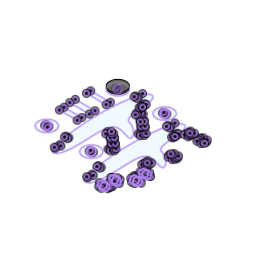
laserbíll (Autodesk Fusion 360 design; units mm, degrees)
Autodesk Fusion 360 part; units mm, degrees
note: some values were not read from the file. Chosen so that the rebuilt part matches the saved one: which bodies a step acts on; which face or edge a step refers to. Set by a fixed rule: which sketch regions a step uses.
(part 1 of 2)
sketch "Sketch2" plane through (0, 0, 0) normal (1, 0, 0) x (0, 1, 0)
  line L0 (0, 0) -> (0, 3) construction
  line L1 (0, 3) -> (-40, 3) construction
  line L2 (-40, 3) -> (-160.4178, 3) construction
  line L3 (-14.8797, 3) -> (-11.8797, 3)
  line L4 (-11.8797, 3) -> (-11.8797, -3)
  line L5 (-14.8797, -3) -> (-14.8797, 3)
  spline S0 degree 5 poles (0, 0) (-0.4976, -0.0964) (-1.4854, -0.3042) (-2.945, -0.6607) (-4.8535, -1.2067) (-7.2026, -1.9204) (-9.0712, -2.4375) (-10.4741, -2.7532) (-11.4109, -2.9243) (-11.8797, -3) knots 0 0 0 0 0 0 0.2 0.4 0.6 0.8 1 1 1 1 1 1
  line L6 (1.6866, 0.3268) -> (-1.6866, -0.3268)
  line L7 (-10.2925, -2.7437) -> (-13.4669, -3.2563)
  line L8 (-160.4178, 3) -> (-163.4178, 3)
  line L9 (-163.4178, 3) -> (-163.4178, -3)
  line L10 (-160.4178, -3) -> (-160.4178, 3)
  spline S1 degree 5 poles (-14.8797, -3) (-22.3096, -4.1508) (-36.7037, -6.1171) (-56.899, -8.0619) (-81.4164, -8.9223) (-109.3682, -8.0716) (-130.3752, -6.4401) (-145.595, -4.8529) (-155.5147, -3.6429) (-160.4178, -3) knots 0 0 0 0 0 0 0.2 0.4 0.6 0.8 1 1 1 1 1 1
  line L11 (2.0883, -0.3719) -> (-31.8477, -5.6281)
  line L12 (-149.202, -4.4707) -> (-171.6337, -1.5293)
  spline S2 degree 5 poles (0, 0) (1.0214, 1.1786) (2.8685, 3.4561) (5.0525, 6.633) (6.7903, 10.3902) (7.0201, 14.2972) (5.3558, 17.4431) (1.9, 19.8865) (-3.1724, 21.7265) (-9.6182, 23.091) (-17.1297, 24.1256) (-25.3371, 24.9813) (-33.8146, 25.8044) (-42.0773, 26.723) (-49.6078, 27.8419) (-55.9536, 29.2551) (-60.806, 31.0538) (-64.092, 33.3377) (-66.0502, 36.222) (-67.344, 39.8538) (-68.8404, 44.3379) (-71.3179, 49.6389) (-75.2304, 55.5069) (-80.3697, 61.3547) (-85.9901, 66.3649) (-91.1225, 69.6901) (-94.8388, 70.6334) (-96.5098, 68.8155) (-96.1359, 64.402) (-94.2949, 58.0341) (-91.8952, 50.6114) (-89.9846, 43.1151) (-89.5511, 36.4298) (-91.2912, 31.1286) (-95.5355, 27.4211) (-102.3274, 25.2561) (-111.4597, 24.382) (-122.527, 24.4246) (-134.9716, 24.9543) (-148.1309, 25.5642) (-161.285, 25.924) (-173.707, 25.7763) (-184.7129, 24.9433) (-193.7115, 23.3296) (-200.2539, 20.9266) (-204.0865, 17.8175) (-205.1955, 14.1795) (-203.8722, 10.294) (-200.7195, 6.5331) (-196.466, 3.2637) (-191.8243, 0.7734) (-187.3088, -0.8279) (-183.1451, -1.6443) (-179.3481, -1.905) (-175.7677, -1.905) (-172.1417, -1.9268) (-168.9623, -2.1457) (-166.3081, -2.4941) (-164.4038, -2.8164) (-163.4178, -3) knots 0 0 0 0 0 0 0.018182 0.036364 0.054545 0.072727 0.090909 0.109091 0.127273 0.145455 0.163636 0.181818 0.2 0.218182 0.236364 0.254545 0.272727 0.290909 0.309091 0.327273 0.345455 0.363636 0.381818 0.4 0.418182 0.436364 0.454545 0.472727 0.490909 0.509091 0.527273 0.545455 0.563636 0.581818 0.6 0.618182 0.636364 0.654545 0.672727 0.690909 0.709091 0.727273 0.745455 0.763636 0.781818 0.8 0.818182 0.836364 0.854545 0.872727 0.890909 0.909091 0.927273 0.945455 0.963636 0.981818 1 1 1 1 1 1
  line L13 (-191.6536, 2.2585) -> (-135.1821, -8.2585)
  line L14 (-184.1519, 9.7365) -> (-194, 8)
  line L15 (-194, 8) -> (-193.4791, 5.0456)
  line L16 (-193.4791, 5.0456) -> (-183.631, 6.7821)
  line L17 (-183.631, 6.7821) -> (-184.1519, 9.7365)
  point P0 (4.968, 17.2018)
  point P1 (-31.0209, 25.5436)
  point P2 (-64.1497, 33.8854)
  point P3 (-72.7298, 51.5223)
  point P4 (-95.1335, 69.6359)
  point P5 (-90, 40)
  point P6 (-131.599, 24.8286)
  point P7 (-204.5301, 15.0567)
  point P8 (-193.3805, 1.7277)
  point P9 (-177.8679, -1.8848)
  dimension "d4" = 3
  dimension "d5" = 3
  dimension "d7" = 3
  dimension "d17" = 6
  dimension "d18" = 6
  dimension "d19" = 6
  dimension "d20" = 6
  dimension "d97" = 10
  dimension "d98" = 3
  constraint coincident L0.start S0.start
  constraint vertical L0
  constraint perpendicular L0 L1
  constraint perpendicular L0 L2
  constraint horizontal L3
  constraint vertical L4
  constraint vertical L5
  constraint coincident L1 L3.start
  constraint midpoint L0.start L6
  constraint midpoint L4.end L7
  constraint horizontal L8
  constraint vertical L9
  constraint vertical L10
  constraint midpoint L5.start L11
  constraint midpoint L10.start L12
  constraint midpoint L9.end L13
  measures "d4" distance of L0.start L0.end
  measures "d5" distance of L3.start L3.end
  measures "d7" distance of L2.end L8.end
  measures "d17" distance of L2.end L10.start
  measures "d18" distance of L8.end L9.end
  measures "d19" distance of L3.start L5.start
  measures "d20" distance of L3.end L4.end
  measures "d97" distance of L14.start L14.end
  measures "d98" distance of L14.start L16.end
extrude "Extrude1" add sketch "Sketch2" along normal blind 3 contours L3 L4 L5 S0 L8 L9 L10 S1 L11 L12 S2 L13 | L4 S0 L11 | L9 L12 L13 makes body 1
sketch "Sketch3" plane through (0, -160.4178, 0) normal (0, -1, 0) x (1, 0, 0)
  line L0 (0, 3) -> (0, -3)
  line L1 (0, -3) -> (3, -3)
  line L2 (3, -3) -> (3, 3)
  line L3 (3, 3) -> (0, 3)
  line L4 (3, 3) -> (9, 3) construction
  line L5 (9, 3) -> (-16, 3)
  line L6 (-16, 3) -> (-16, 0)
  line L7 (-11, -3) -> (9, -3)
  line L8 (9, -3) -> (9, 3)
  line L9 (9, 3) -> (-16, 3)
  line L10 (-16, 3) -> (-16, 6)
  line L11 (-11, 9) -> (9, 9)
  line L12 (9, 9) -> (9, 3)
  line L13 (3, 9) -> (0, 9)
  line L14 (0, 9) -> (0, 3)
  line L15 (0, 3) -> (3, 3)
  line L16 (3, 3) -> (3, 9)
  line L17 (0, 3) -> (-11, 3) construction
  line L18 (-11, 3) -> (-11, 0) construction
  line L19 (-11, 0) -> (-16, 0)
  line L20 (-16, 0) -> (-16, 6)
  line L21 (-16, 6) -> (-11, 6)
  line L22 (-11, 6) -> (-11, 0)
  line L23 (-11, 6) -> (-11, 9)
  line L24 (-11, 0) -> (-11, -4)
  line L25 (-11, 0) -> (-11, -3)
  dimension "d11" = 6
  dimension "d12" = 25
  dimension "d13" = 6
  dimension "d27" = 3
  dimension "d28" = 5
  dimension "d29" = 6
  constraint coincident L2.end L3.start
  constraint perpendicular L2 L4
  constraint horizontal L5
  constraint vertical L6
  constraint horizontal L7
  constraint vertical L8
  constraint horizontal L9
  constraint vertical L10
  constraint horizontal L11
  constraint vertical L12
  constraint horizontal L13
  constraint vertical L14
  constraint horizontal L15
  constraint vertical L16
  constraint coincident L0.start L3.end
  constraint coincident L11 L13.start
  constraint perpendicular L10 L17
  constraint perpendicular L7 L18
  constraint horizontal L19
  constraint vertical L20
  constraint horizontal L21
  constraint vertical L22
  constraint perpendicular L11 L23
  constraint perpendicular L19 L24
  constraint coincident L24 L7.start
  measures "d11" distance of L2.end L4.end
  measures "d12" distance of L4.end L5.end
  measures "d13" distance of L4.end L7.end
  measures "d27" distance of L17.end L18.end
  measures "d28" distance of L18.end L6.end
  measures "d29" distance of L18.end L21.end
extrude "Extrude2" add sketch "Sketch3" along normal blind 3 separate body contours L0 L1 L2 L3 L5 L7 L9 L15 | L0 L5 L7 L9 L22 L24 L25 | L5 L9 L11 L14 L22 L23 | L2 L5 L7 L8 L9 | L5 L9 L11 L12 L16 | L5 L6 L9 L19 L20 L22 | L5 L9 L10 L20 L21 L22 makes body 2
sketch "Sketch4" plane through (0, -11.8797, 0) normal (0, -1, 0) x (1, 0, 0)
  line L0 (0, 3) -> (0, -3)
  line L1 (0, -3) -> (3, -3)
  line L2 (3, -3) -> (3, 3)
  line L3 (3, 3) -> (0, 3)
  line L4 (3, 3) -> (9, 3) construction
  line L5 (9, 3) -> (-21, 3)
  line L6 (-21, 3) -> (-21, 0)
  line L7 (-16, -3) -> (9, -3)
  line L8 (9, -3) -> (9, 3)
  line L9 (-21, 3) -> (9, 3)
  line L10 (9, 3) -> (9, 9)
  line L11 (9, 9) -> (-16, 9)
  line L12 (-21, 6) -> (-21, 3)
  line L13 (3, 9) -> (0, 9)
  line L14 (0, 9) -> (0, 3)
  line L15 (0, 3) -> (3, 3)
  line L16 (3, 3) -> (3, 9)
  line L17 (-21, 6) -> (-16, 6)
  line L18 (-16, 6) -> (-16, 9)
  line L19 (-16, 0) -> (-21, 0)
  line L20 (-16, -3) -> (-16, 0)
  dimension "d21" = 6
  dimension "d22" = 30
  dimension "d23" = 6
  dimension "d41" = 5
  dimension "d42" = 5
  dimension "d114" = 25
  constraint coincident L2.end L3.start
  constraint perpendicular L2 L4
  constraint horizontal L5
  constraint vertical L6
  constraint horizontal L7
  constraint vertical L8
  constraint horizontal L9
  constraint vertical L10
  constraint horizontal L11
  constraint vertical L12
  constraint horizontal L13
  constraint vertical L14
  constraint horizontal L15
  constraint vertical L16
  constraint coincident L0.start L3.end
  constraint coincident L11 L13.start
  constraint horizontal L17
  constraint vertical L18
  constraint horizontal L19
  constraint vertical L20
  measures "d21" distance of L2.end L4.end
  measures "d22" distance of L4.end L5.end
  measures "d23" distance of L4.end L7.end
  measures "d41" distance of L19.start L6.end
  measures "d42" distance of L12.start L17.end
  measures "d114" distance of L10.end L11.end
extrude "Extrude3" add sketch "Sketch4" along normal blind 3 separate body contours L0 L1 L2 L3 L5 L7 L9 L15 | L0 L5 L6 L7 L9 L19 L20 | L5 L9 L11 L12 L14 L17 L18 | L2 L5 L7 L8 L9 | L5 L9 L10 L11 L16 makes body 3
sketch "Sketch5" plane through (-16, 0, 0) normal (-1, 0, 0) x (0, -1, 0)
  line L0 (160.4178, 6) -> (160.4178, 0)
  line L1 (160.4178, 0) -> (163.4178, 0)
  line L2 (163.4178, 0) -> (163.4178, 6)
  line L3 (163.4178, 6) -> (160.4178, 6)
  line L4 (160.4178, 6) -> (160.4178, 3) construction
  circle A0 centre (161.9178, 3) radius 17.5
  line L5 (160.4178, 6) -> (163.4178, 6)
  line L6 (163.4178, 6) -> (163.4178, 0)
  line L7 (163.4178, 0) -> (160.4178, 0)
  line L8 (160.4178, 0) -> (160.4178, 6)
  dimension "d31" = 35
  dimension "d38" = 1.5
  constraint coincident L0.start L3.end
  constraint midpoint L0 L4.end
  constraint horizontal L5
  constraint vertical L6
  constraint horizontal L7
  constraint vertical L8
  constraint coincident L1.end L2.start
  measures "d31" diameter of A0
  measures "d38" distance of L4.end A0.centre
sketch "Sketch6" plane through (-21, 0, 0) normal (-1, 0, 0) x (0, -1, 0)
  line L0 (11.8797, 6) -> (11.8797, 0)
  line L1 (11.8797, 0) -> (14.8797, 0)
  line L2 (14.8797, 0) -> (14.8797, 6)
  line L3 (14.8797, 6) -> (11.8797, 6)
  line L4 (11.8797, 6) -> (11.8797, 3)
  line L5 (11.8797, 3) -> (13.3797, 3)
  circle A0 centre (13.3797, 3) radius 17.5
  line L6 (11.8797, 6) -> (14.8797, 6)
  line L7 (14.8797, 6) -> (14.8797, 0)
  line L8 (14.8797, 0) -> (11.8797, 0)
  line L9 (11.8797, 0) -> (11.8797, 6)
  dimension "d35" = 1.5
  dimension "d37" = 35
  constraint coincident L0.start L3.end
  constraint perpendicular L3 L4
  constraint coincident L5.end A0.centre
  constraint vertical L7
  constraint horizontal L8
  constraint coincident L1.end L2.start
  measures "d35" distance of L4.end L5.end
  measures "d37" diameter of A0
extrude "Extrude4" add sketch "Sketch5" against normal blind 3 separate body makes body 4
extrude "Extrude12" add sketch "Sketch6" against normal blind 3 separate body makes body 5
sketch "Sketch7" plane through (0, 0, 0) normal (-1, 0, 0) x (0, -1, 0)
  line L0 (14.8797, 3) -> (14.8797, -3)
  spline S0 degree 5 poles (14.8797, -3) (22.3096, -4.1508) (36.7037, -6.1171) (56.899, -8.0619) (81.4164, -8.9223) (109.3682, -8.0716) (130.3752, -6.4401) (145.595, -4.8529) (155.5147, -3.6429) (160.4178, -3) knots 0 0 0 0 0 0 0.2 0.4 0.6 0.8 1 1 1 1 1 1
  line L1 (160.4178, -3) -> (160.4178, 3)
  line L2 (160.4178, 3) -> (163.4178, 3)
  line L3 (163.4178, 3) -> (163.4178, -3)
  spline S1 degree 5 poles (0, 0) (-1.0214, 1.1786) (-2.8685, 3.4561) (-5.0525, 6.633) (-6.7903, 10.3902) (-7.0201, 14.2972) (-5.3558, 17.4431) (-1.9, 19.8865) (3.1724, 21.7265) (9.6182, 23.091) (17.1297, 24.1256) (25.3371, 24.9813) (33.8146, 25.8044) (42.0773, 26.723) (49.6078, 27.8419) (55.9536, 29.2551) (60.806, 31.0538) (64.092, 33.3377) (66.0502, 36.222) (67.344, 39.8538) (68.8404, 44.3379) (71.3179, 49.6389) (75.2304, 55.5069) (80.3697, 61.3547) (85.9901, 66.3649) (91.1225, 69.6901) (94.8388, 70.6334) (96.5098, 68.8155) (96.1359, 64.402) (94.2949, 58.0341) (91.8952, 50.6114) (89.9846, 43.1151) (89.5511, 36.4298) (91.2912, 31.1286) (95.5355, 27.4211) (102.3274, 25.2561) (111.4597, 24.382) (122.527, 24.4246) (134.9716, 24.9543) (148.1309, 25.5642) (161.285, 25.924) (173.707, 25.7763) (184.7129, 24.9433) (193.7115, 23.3296) (200.2539, 20.9266) (204.0865, 17.8175) (205.1955, 14.1795) (203.8722, 10.294) (200.7195, 6.5331) (196.466, 3.2637) (191.8243, 0.7734) (187.3088, -0.8279) (183.1451, -1.6443) (179.3481, -1.905) (175.7677, -1.905) (172.1417, -1.9268) (168.9623, -2.1457) (166.3081, -2.4941) (164.4038, -2.8164) (163.4178, -3) knots 0 0 0 0 0 0 0.018182 0.036364 0.054545 0.072727 0.090909 0.109091 0.127273 0.145455 0.163636 0.181818 0.2 0.218182 0.236364 0.254545 0.272727 0.290909 0.309091 0.327273 0.345455 0.363636 0.381818 0.4 0.418182 0.436364 0.454545 0.472727 0.490909 0.509091 0.527273 0.545455 0.563636 0.581818 0.6 0.618182 0.636364 0.654545 0.672727 0.690909 0.709091 0.727273 0.745455 0.763636 0.781818 0.8 0.818182 0.836364 0.854545 0.872727 0.890909 0.909091 0.927273 0.945455 0.963636 0.981818 1 1 1 1 1 1
  spline S2 degree 5 poles (0, 0) (0.4976, -0.0964) (1.4854, -0.3042) (2.945, -0.6607) (4.8535, -1.2067) (7.2026, -1.9204) (9.0712, -2.4375) (10.4741, -2.7532) (11.4109, -2.9243) (11.8797, -3) knots 0 0 0 0 0 0 0.2 0.4 0.6 0.8 1 1 1 1 1 1
  line L4 (11.8797, -3) -> (11.8797, 3)
  line L5 (11.8797, 3) -> (14.8797, 3)
  line L6 (16.2787, 23.9531) -> (29.2024, 25.3596)
  line L7 (16.2787, 23.9531) -> (20.5866, 24.422)
  line L8 (29.2024, 25.3596) -> (24.8945, 24.8908)
  line L9 (16.2787, 23.9531) -> (16.6033, 20.9707)
  line L10 (16.6033, 20.9707) -> (20.9112, 21.4396)
  line L11 (20.9112, 21.4396) -> (20.5866, 24.422)
  line L12 (24.8945, 24.8908) -> (25.2191, 21.9084)
  line L13 (25.2191, 21.9084) -> (29.527, 22.3772)
  line L14 (29.527, 22.3772) -> (29.2024, 25.3596)
  line L15 (24.8945, 24.8908) -> (29.2024, 25.3596)
  line L16 (28.6636, 30.3105) -> (24.8945, 26.013)
  line L17 (24.8945, 26.013) -> (24.8945, 24.8908)
  line L18 (28.6636, 30.3105) -> (29.2024, 25.3596)
  line L19 (20.5866, 24.422) -> (20.4846, 25.3596)
  line L20 (20.4846, 25.3596) -> (16.1767, 24.8908)
  line L21 (16.1767, 24.8908) -> (16.2787, 23.9531)
  line L22 (183.631, 6.7821) -> (184.1519, 9.7365)
  line L23 (184.1519, 9.7365) -> (194, 8)
  line L24 (194, 8) -> (193.4791, 5.0456)
  line L25 (193.4791, 5.0456) -> (183.631, 6.7821)
  dimension "d43" = 13
  dimension "d44" = 4.3333
  dimension "d45" = 4.3333
  dimension "d46" = 3
  dimension "d47" = 4.3333
  dimension "d48" = 3
  dimension "d49" = 4.3333
  constraint coincident S1 L6.start
  constraint parallel L6 L7
  constraint parallel L6 L8
  constraint perpendicular L6 L9
  constraint perpendicular L9 L10
  constraint perpendicular L6 L12
  constraint perpendicular L12 L13
  constraint vertical L17
  constraint perpendicular L15 L18
  constraint perpendicular L7 L19
  constraint perpendicular L19 L20
  constraint perpendicular L6 L21
  measures "d43" distance of L6.start L6.end
  measures "d44" distance of L6.start L7.end
  measures "d45" distance of L6.end L8.end
  measures "d46" distance of L6.start L9.end
  measures "d47" distance of L9.end L10.end
  measures "d48" distance of L8.end L12.end
  measures "d49" distance of L12.end L13.end
extrude "Extrude5" cut sketch "Sketch7" against normal blind 3 contours S1 L19 L20 L21 | S1 L6 L7 L19 | L6 L7 L9 L10 L11 | S1 L6 L8 L15 L17 | L6 L8 L12 L13 L14 L15 | S1 L16 L17 L18 bodies 1
sketch "Sketch8" plane through (0, 0, 0) normal (-1, 0, 0) x (0, -1, 0)
  line L0 (20.5823, 24.4619) -> (20.9112, 21.4396)
  line L1 (20.9112, 21.4396) -> (16.6033, 20.9707)
  line L2 (16.6033, 20.9707) -> (16.2787, 23.9531)
  spline S0 degree 5 poles (0, 0) (-1.0214, 1.1786) (-2.8685, 3.4561) (-5.0525, 6.633) (-6.7903, 10.3902) (-7.0201, 14.2972) (-5.3558, 17.4431) (-1.9, 19.8865) (3.0388, 21.678) (7.9907, 22.7458) (12.1064, 23.3992) (14.9359, 23.7825) (16.2787, 23.9531) knots 0 0 0 0 0 0 0.018182 0.036364 0.054545 0.072727 0.090909 0.109091 0.127273 0.14306 0.14306 0.14306 0.14306 0.14306 0.14306
  spline S1 degree 5 poles (0, 0) (0.4976, -0.0964) (1.4854, -0.3042) (2.945, -0.6607) (4.8535, -1.2067) (7.2026, -1.9204) (9.0712, -2.4375) (10.4741, -2.7532) (11.4109, -2.9243) (11.8797, -3) knots 0 0 0 0 0 0 0.2 0.4 0.6 0.8 1 1 1 1 1 1
  line L3 (11.8797, -3) -> (11.8797, 3)
  line L4 (11.8797, 3) -> (14.8797, 3)
  line L5 (14.8797, 3) -> (14.8797, -3)
  spline S2 degree 5 poles (14.8797, -3) (22.3096, -4.1508) (36.7037, -6.1171) (56.899, -8.0619) (81.4164, -8.9223) (109.3682, -8.0716) (130.3752, -6.4401) (145.595, -4.8529) (155.5147, -3.6429) (160.4178, -3) knots 0 0 0 0 0 0 0.2 0.4 0.6 0.8 1 1 1 1 1 1
  line L6 (160.4178, -3) -> (160.4178, 3)
  line L7 (160.4178, 3) -> (163.4178, 3)
  line L8 (163.4178, 3) -> (163.4178, -3)
  spline S3 degree 5 poles (29.2025, 25.3586) (30.1153, 25.451) (32.7052, 25.7143) (36.9634, 26.1574) (42.7626, 26.8248) (49.6078, 27.8419) (55.9536, 29.2551) (60.806, 31.0538) (64.092, 33.3377) (66.0502, 36.222) (67.344, 39.8538) (68.8404, 44.3379) (71.3179, 49.6389) (75.2304, 55.5069) (80.3697, 61.3547) (85.9901, 66.3649) (91.1225, 69.6901) (94.8388, 70.6334) (96.5098, 68.8155) (96.1359, 64.402) (94.2949, 58.0341) (91.8952, 50.6114) (89.9846, 43.1151) (89.5511, 36.4298) (91.2912, 31.1286) (95.5355, 27.4211) (102.3274, 25.2561) (111.4597, 24.382) (122.527, 24.4246) (134.9716, 24.9543) (148.1309, 25.5642) (161.285, 25.924) (173.707, 25.7763) (184.7129, 24.9433) (193.7115, 23.3296) (200.2539, 20.9266) (204.0865, 17.8175) (205.1955, 14.1795) (203.8722, 10.294) (200.7195, 6.5331) (196.466, 3.2637) (191.8243, 0.7734) (187.3088, -0.8279) (183.1451, -1.6443) (179.3481, -1.905) (175.7677, -1.905) (172.1417, -1.9268) (168.9623, -2.1457) (166.3081, -2.4941) (164.4038, -2.8164) (163.4178, -3) knots 0.171909 0.171909 0.171909 0.171909 0.171909 0.171909 0.181818 0.2 0.218182 0.236364 0.254545 0.272727 0.290909 0.309091 0.327273 0.345455 0.363636 0.381818 0.4 0.418182 0.436364 0.454545 0.472727 0.490909 0.509091 0.527273 0.545455 0.563636 0.581818 0.6 0.618182 0.636364 0.654545 0.672727 0.690909 0.709091 0.727273 0.745455 0.763636 0.781818 0.8 0.818182 0.836364 0.854545 0.872727 0.890909 0.909091 0.927273 0.945455 0.963636 0.981818 1 1 1 1 1 1
  line L9 (29.2025, 25.3586) -> (29.527, 22.3772)
  line L10 (29.527, 22.3772) -> (25.2191, 21.9084)
  line L11 (25.2191, 21.9084) -> (24.8945, 24.8908)
  line L12 (24.8945, 24.8908) -> (24.8945, 24.9206)
  spline S4 degree 5 poles (20.5823, 24.4619) (21.4324, 24.5563) (22.2898, 24.649) (23.1533, 24.7403) (24.0219, 24.8308) (24.8945, 24.9206) knots 0.152948 0.152948 0.152948 0.152948 0.152948 0.152948 0.162519 0.162519 0.162519 0.162519 0.162519 0.162519
  line L13 (16.6033, 20.9707) -> (17.1253, 21.0275)
  line L14 (20.9112, 21.4396) -> (20.5823, 24.4619)
  line L15 (20.5823, 24.4619) -> (24.8945, 24.9206)
  line L16 (25.2191, 21.9084) -> (24.8945, 24.9206)
  line L17 (25.2191, 21.9084) -> (29.527, 22.3772)
  line L18 (29.527, 22.3772) -> (29.2025, 25.3586)
  line L19 (29.2025, 25.3586) -> (28.6615, 30.3292)
  line L20 (15.7379, 28.9227) -> (16.6034, 20.9697)
  line L21 (15.7379, 28.9227) -> (20.0458, 29.3915)
  line L22 (20.0458, 29.3915) -> (20.3703, 26.4091)
  line L23 (20.3703, 26.4091) -> (24.6782, 26.878)
  line L24 (24.6782, 26.878) -> (24.3536, 29.8604)
  line L25 (28.6615, 30.3292) -> (24.3536, 29.8604)
  line L26 (20.0458, 29.3915) -> (15.7379, 28.9227)
  line L27 (183.631, 6.7821) -> (184.1519, 9.7365)
  line L28 (184.1519, 9.7365) -> (194, 8)
  line L29 (194, 8) -> (193.4791, 5.0456)
  line L30 (193.4791, 5.0456) -> (183.631, 6.7821)
  dimension "d52" = 5
  dimension "d53" = 13
  dimension "d54" = 8
  dimension "d55" = 4.3333
  dimension "d56" = 3
  dimension "d57" = 4.3333
  constraint coincident L1.end L2.start
  constraint coincident L1 L13.end
  constraint perpendicular L2 L13
  constraint coincident L0.end L1.start
  constraint coincident L0.start S4.start
  constraint coincident L12.end S4.end
  constraint coincident L10.end L11.start
  constraint coincident L9.end L10.start
  constraint coincident S3.start L9.start
  constraint perpendicular L10 L19
  constraint perpendicular L19 L25
  constraint perpendicular L1 L20
  constraint perpendicular L20 L21
  constraint perpendicular L21 L22
  constraint perpendicular L22 L23
  constraint perpendicular L24 L25
  constraint collinear L25 L26
  measures "d52" distance of S3.start L19.end
  measures "d53" distance of L19.end L20.start
  measures "d54" distance of L20.start L20.end
  measures "d55" distance of L20.start L21.end
  measures "d56" distance of L21.end L22.end
  measures "d57" distance of L22.end L23.end
extrude "Extrude6" add sketch "Sketch8" against normal blind 3 separate body contours L0 L1 L2 L9 L10 S4 L13 L14 L16 L17 L18 L19 L20 L21 L22 L23 L24 L25 L26 makes body 6
sketch "Sketch9" plane through (0, 2.9266, 26.8914) normal (0, 0.108193, 0.99413) x (-1, 0, 0)
  line L0 (0, 18.7747) -> (0, 23.108)
  line L1 (0, 23.108) -> (-3, 23.108)
  line L2 (-3, 23.108) -> (-3, 18.7747)
  line L3 (-3, 18.7747) -> (0, 18.7747)
  line L4 (0, 18.7747) -> (0, 23.108)
  line L5 (0, 23.108) -> (-3, 23.108)
  line L6 (-3, 23.108) -> (-3, 27.4414)
  line L7 (-3, 27.4414) -> (0, 27.4414)
  line L8 (0, 27.4414) -> (0, 31.7747)
  line L9 (0, 31.7747) -> (9, 31.7747)
  line L10 (12, 27.4414) -> (12, 23.108)
  line L11 (9, 18.7747) -> (0, 18.7747)
  line L12 (9, 18.7747) -> (9, 23.108)
  line L13 (9, 23.108) -> (12, 23.108)
  line L14 (12, 23.108) -> (12, 27.4414) construction
  line L15 (12, 27.4414) -> (9, 27.4414)
  line L16 (9, 27.4414) -> (9, 31.7747)
  dimension "d60" = 4.3333
  dimension "d61" = 3
  dimension "d62" = 4.3333
  dimension "d63" = 3
  dimension "d64" = 4.3333
  dimension "d71" = 4.3333
  dimension "d72" = 3
  dimension "d76" = 9
  dimension "d77" = 9
  constraint coincident L0.start L3.end
  constraint perpendicular L1 L4
  constraint coincident L1.end L2.start
  constraint perpendicular L5 L6
  constraint perpendicular L6 L7
  constraint perpendicular L7 L8
  constraint perpendicular L8 L9
  constraint perpendicular L9 L10
  constraint perpendicular L0 L11
  constraint vertical L12
  constraint horizontal L13
  constraint perpendicular L13 L14
  constraint horizontal L15
  constraint vertical L16
  measures "d60" distance of L0.start L0.end
  measures "d61" distance of L0.end L1.end
  measures "d62" distance of L1.end L6.end
  measures "d63" distance of L6.end L7.end
  measures "d64" distance of L7.end L8.end
  measures "d71" distance of L10.end L10.start
  measures "d72" distance of L10.start L15.end
  measures "d76" distance of L8.end L9.end
  measures "d77" distance of L0.start L11.start
extrude "Extrude7" add sketch "Sketch9" against normal blind 3 separate body contours L0 L1 L4 L5 L6 L7 L8 L9 L10 L11 L12 L13 L15 L16 makes body 7
sketch "Sketch10" plane through (-9, 0, 0) normal (-1, 0, 0) x (0, -1, 0)
  line L0 (20.0458, 29.3915) -> (15.7379, 28.9227)
  line L1 (15.7379, 28.9227) -> (16.0624, 25.9403)
  line L2 (16.0624, 25.9403) -> (20.3703, 26.4091)
  line L3 (20.3703, 26.4091) -> (20.0458, 29.3915)
  line L4 (16.0624, 25.9403) -> (20.3703, 26.4091)
  line L5 (20.3703, 26.4091) -> (20.0458, 29.3915)
  line L6 (20.0458, 29.3915) -> (24.3536, 29.8604)
  line L7 (24.3536, 29.8604) -> (24.6782, 26.878)
  line L8 (24.6782, 26.878) -> (29.6489, 27.4189)
  line L9 (20.3703, 26.4091) -> (7.4466, 25.0026)
  line L10 (-0.2696, 31.2042) -> (-0.9188, 37.169)
  line L11 (35.8504, 35.1352) -> (35.2013, 41.1)
  line L12 (27.485, 47.3015) -> (5.2828, 44.8852)
  arc A0 (5.2828, 44.8852) -> (-0.9188, 37.169) centre (6.0401, 37.9263) ccw
  arc A1 (35.2013, 41.1) -> (27.485, 47.3015) centre (28.2424, 40.3426) ccw
  arc A2 (29.6489, 27.4189) -> (35.8504, 35.1352) centre (28.8915, 34.3779) ccw
  arc A3 (-0.2696, 31.2042) -> (7.4466, 25.0026) centre (6.6893, 31.9616) ccw
  line L13 (6.0401, 37.9263) -> (11.5247, 37.9263)
  line L14 (5.1011, 43.3756) -> (15.4934, 37.3756)
  line L15 (15.4934, 37.3756) -> (13.9934, 34.7775)
  line L16 (13.9934, 34.7775) -> (3.6011, 40.7775)
  line L17 (3.6011, 40.7775) -> (5.1011, 43.3756)
  line L18 (3.6011, 40.7775) -> (12.5508, 40.7775) construction
  line L19 (19, 35) -> (28, 35)
  line L20 (28, 35) -> (28, 32)
  line L21 (28, 32) -> (19, 32)
  line L22 (19, 32) -> (19, 35)
  point P0 (36.6078, 28.1763)
  point P1 (0.4877, 24.2453)
  point P2 (-1.6761, 44.1279)
  point P3 (34.4439, 48.0589)
  dimension "d80" = 4.3333
  dimension "d81" = 3
  dimension "d82" = 12
  dimension "d83" = 20
  dimension "d84" = 20
  dimension "d85" = 20
  dimension "d86" = 7
  dimension "d87" = 12
  dimension "d88" = 3
  dimension "d89" = 12
  dimension "d90" = 60
  dimension "d91" = 3
  dimension "d92" = 3
  dimension "d93" = 9
  dimension "d94" = 3
  constraint coincident L1.end L2.start
  constraint coincident L2.end L3.start
  constraint coincident L0.start L3.end
  constraint perpendicular L5 L6
  constraint perpendicular L6 L7
  constraint perpendicular L7 L8
  constraint perpendicular L1 L9
  constraint perpendicular L9 L10
  constraint perpendicular L8 L11
  constraint coincident P2 L10
  constraint coincident P2 L12
  constraint tangent L10 A0
  constraint tangent L12 A0
  constraint coincident P3 L11
  constraint coincident P3 L12
  constraint tangent L11 A1
  constraint tangent L12 A1
  constraint equal A0 A1
  constraint coincident P0 L8
  constraint coincident P0 L11
  constraint tangent L8 A2
  constraint tangent L11 A2
  constraint equal A0 A2
  constraint coincident P1 L9
  constraint coincident P1 L10
  constraint tangent L9 A3
  constraint tangent L10 A3
  constraint equal A0 A3
  constraint coincident A0.centre L13.start
  constraint horizontal L13
  constraint perpendicular L14 L15
  constraint perpendicular L15 L16
  constraint horizontal L18
  constraint perpendicular L14 L17
  constraint horizontal L19
  constraint perpendicular L19 L20
  constraint perpendicular L20 L21
  constraint perpendicular L19 L22
  measures "d80" distance of L0.start L6.end
  measures "d81" distance of L6.end L7.end
  measures "d82" distance of L7.end P0
  measures "d83" distance of L2.end P1
  measures "d84" distance of P1 P2
  measures "d85" distance of P0 P3
  measures "d86" radius of A0
  measures "d87" distance of L14.start L14.end
  measures "d88" distance of L14.end L15.end
  measures "d89" distance of L15.end L16.end
  measures "d90" angle of L17 L18
  measures "d91" distance of L14.start L16.end
  measures "d92" distance of L19.end L20.end
  measures "d93" distance of L20.end L21.end
  measures "d94" distance of L21.end L19.start
extrude "Extrude8" add sketch "Sketch10" along normal blind 3 separate body makes body 8
sketch "Sketch11" plane through (0, 0, 0) normal (1, 0, 0) x (0, 1, 0)
sketch "Sketch12" plane through (0, -6.697, 37.9803) normal (0, -0.173648, 0.984808) x (1, 0, 0)
  line L0 (0, -179.6635) -> (0, -189.6635)
  line L1 (0, -189.6635) -> (3, -189.6635)
  line L2 (3, -189.6635) -> (3, -179.6635)
  line L3 (3, -179.6635) -> (0, -179.6635)
  line L4 (0, -179.6635) -> (-10, -179.6635)
  line L5 (-10, -179.6635) -> (-10, -189.6635)
  line L6 (-10, -189.6635) -> (9, -189.6635)
  line L7 (9, -189.6635) -> (9, -179.6635)
  line L8 (9, -179.6635) -> (0, -179.6635)
  dimension "d99" = 10
  dimension "d100" = 10
  dimension "d101" = 19
  dimension "d102" = 10
  constraint coincident L0.start L3.end
  constraint perpendicular L0 L4
  constraint perpendicular L4 L5
  constraint perpendicular L2 L6
  constraint perpendicular L6 L7
  measures "d99" distance of L0.start L4.end
  measures "d100" distance of L4.end L5.end
  measures "d101" distance of L5.end L6.end
  measures "d102" distance of L6.end L7.end
extrude "Extrude9" add sketch "Sketch12" along normal blind 3 separate body makes body 9
sketch "Sketch13" plane through (0, -18.5574, 32.1424) normal (0, -0.5, 0.866025) x (1, 0, 0)
  line L0 (-9, 5.2701) -> (-9, 17.2701)
  line L1 (-9, 17.2701) -> (-12, 17.2701)
  line L2 (-12, 17.2701) -> (-12, 5.2701)
  line L3 (-12, 5.2701) -> (-9, 5.2701)
  line L4 (-12, 17.2701) -> (9, 17.2701)
  line L5 (-12, 17.2701) -> (-12, 5.2701)
  line L6 (-12, 5.2701) -> (9, 5.2701)
  line L7 (9, 5.2701) -> (9, 17.2701)
  dimension "d105" = 21
  dimension "d106" = 21
  constraint coincident L1.end L2.start
  constraint perpendicular L0 L4
  constraint coincident L2.end L3.start
  constraint perpendicular L5 L6
  measures "d105" distance of L1.end L4.end
  measures "d106" distance of L2.end L6.end
extrude "Extrude10" add sketch "Sketch13" along normal blind 3 separate body makes body 10
sketch "Sketch14" plane through (0, 0, 32) normal (0, 0, 1) x (-1, 0, 0)
  line L0 (9, 28) -> (9, 19)
  line L1 (9, 19) -> (12, 19)
  line L2 (12, 19) -> (12, 28)
  line L3 (12, 28) -> (9, 28)
  line L4 (12, 19) -> (-9, 19)
  line L5 (-9, 19) -> (-9, 28)
  line L6 (-9, 28) -> (12, 28)
  line L7 (12, 28) -> (12, 19)
  dimension "d109" = 21
  dimension "d110" = 9
  constraint horizontal L4
  constraint vertical L5
  constraint horizontal L6
  constraint vertical L7
  constraint coincident L1.end L2.start
  measures "d109" distance of L1.end L4.end
  measures "d110" distance of L1.end L2.end
extrude "Extrude11" add sketch "Sketch14" along normal blind 3 separate body makes body 11
ref_plane "WorkPlane1" through (9, 0, 0) normal (1, 0, 0) x (0, 1, 0)
mirror "Mirror3" about plane through (9, 0, 0) normal (1, 0, 0) of bodies 11 7 2 5 8 10 6 9 1 4 3 makes body 12 at (18, -96.574, 3.4974) makes body 13 at (23.3333, -11.8797, 6) makes body 14 at (25.3333, -160.4178, 3) makes body 15 at (34, -155.0845, 3) makes body 16 at (15, -27.5141, 27.5219) makes body 17 at (24, -22.9177, 29.7041) makes body 18 at (27, -16.0871, 43.1874) makes body 19 at (24.6667, -190.1964, 5.6244) makes body 20 at (21, -7.0652, 38.7775) makes body 21 at (15, -25, 32) makes body 22 at (39, -20.2131, 3)
combine "Combine6" operation add target body 20 tool bodies 10
combine "Combine7" operation add target body 21 tool bodies 11
combine "Combine8" operation add target body 3 tool bodies 13
combine "Combine9" operation add target body 2 tool bodies 14
combine "Combine10" operation add target body 9 tool bodies 19
copy_body "Body->Comp20" bodies 5 removing the originals makes body 23 in component "hægra afturhjól (1)"
copy_body "Body->Comp21" bodies 9 removing the originals makes body 24 in component "framvængur"
copy_body "Body->Comp22" bodies 2 removing the originals makes body 25 in component "framöxull"
copy_body "Body->Comp23" bodies 3 removing the originals makes body 26 in component "Component''''"
copy_body "Body->Comp24" bodies 12 removing the originals makes body 27 in component "Body hægri (1)"
copy_body "Body->Comp25" bodies 15 removing the originals makes body 28 in component "hægra afturhjól (2)"
copy_body "Body->Comp26" bodies 16 removing the originals makes body 29 in component "hægri afturvængsfesting1 (1)"
copy_body "Body->Comp27" bodies 17 removing the originals makes body 30 in component "hægri afturvængsfesting 2 (1)"
copy_body "Body->Comp28" bodies 18 removing the originals makes body 31 in component "hægri hliðaplata (1)"
copy_body "Body->Comp29" bodies 20 removing the originals makes body 32 in component "afturvængur efri (1)"
copy_body "Body->Comp30" bodies 21 removing the originals makes body 33 in component "afturvængur neðri (1)"
copy_body "Body->Comp31" bodies 22 removing the originals makes body 34 in component "hægra afturhjól (1) (1)"
copy_body "Body->Comp32" bodies 8 removing the originals makes body 35 in component "hægri hliðaplata"
copy_body "Body->Comp33" bodies 7 removing the originals makes body 36 in component "hægri afturvængsfesting 2"
copy_body "Body->Comp34" bodies 6 removing the originals makes body 37 in component "hægri afturvængsfesting1"
copy_body "Body->Comp35" bodies 4 removing the originals makes body 38 in component "hægra afturhjól"
copy_body "Body->Comp36" bodies 1 removing the originals makes body 39 in component "Body hægri"
sketch "Sketch16" plane through (0, 0, 0) normal (0, 0, 1) x (1, 0, 0)
  line L0 (-67.9483, -40.5823) -> (-70.9706, -40.9112)
  line L1 (-70.9706, -40.9112) -> (-71.4395, -36.6033)
  line L2 (-71.4395, -36.6033) -> (-68.4571, -36.2787)
  spline S0 degree 5 poles (-92.4102, -20) (-91.2316, -18.9786) (-88.9541, -17.1315) (-85.7772, -14.9475) (-82.02, -13.2097) (-78.113, -12.9799) (-74.9671, -14.6442) (-72.5237, -18.1) (-70.7322, -23.0388) (-69.6644, -27.9907) (-69.011, -32.1064) (-68.6277, -34.9359) (-68.4571, -36.2787) knots 0 0 0 0 0 0 0.018182 0.036364 0.054545 0.072727 0.090909 0.109091 0.127273 0.14306 0.14306 0.14306 0.14306 0.14306 0.14306
  spline S1 degree 5 poles (-95.4102, -31.8797) (-95.3345, -31.4109) (-95.1634, -30.4741) (-94.8477, -29.0712) (-94.3306, -27.2026) (-93.6169, -24.8535) (-93.0709, -22.945) (-92.7144, -21.4854) (-92.5066, -20.4976) (-92.4102, -20) knots -1 -1 -1 -1 -1 -1 -0.8 -0.6 -0.4 -0.2 0 0 0 0 0 0
  line L3 (-95.4102, -31.8797) -> (-89.4102, -31.8797)
  line L4 (-89.4102, -31.8797) -> (-89.4102, -34.8797)
  line L5 (-89.4102, -34.8797) -> (-95.4102, -34.8797)
  spline S2 degree 5 poles (-95.4102, -180.4178) (-96.0531, -175.5147) (-97.2631, -165.595) (-98.8503, -150.3752) (-100.4818, -129.3682) (-101.3325, -101.4164) (-100.4721, -76.899) (-98.5273, -56.7037) (-96.561, -42.3096) (-95.4102, -34.8797) knots -1 -1 -1 -1 -1 -1 -0.8 -0.6 -0.4 -0.2 0 0 0 0 0 0
  line L6 (-95.4102, -180.4178) -> (-89.4102, -180.4178)
  line L7 (-89.4102, -180.4178) -> (-89.4102, -183.4178)
  line L8 (-89.4102, -183.4178) -> (-95.4102, -183.4178)
  spline S3 degree 5 poles (-67.0516, -49.2025) (-66.9592, -50.1153) (-66.6959, -52.7052) (-66.2528, -56.9634) (-65.5854, -62.7626) (-64.5683, -69.6078) (-63.1551, -75.9536) (-61.3564, -80.806) (-59.0725, -84.092) (-56.1882, -86.0502) (-52.5564, -87.344) (-48.0722, -88.8404) (-42.7713, -91.3179) (-36.9033, -95.2304) (-31.0555, -100.3697) (-26.0453, -105.9901) (-22.7201, -111.1225) (-21.7768, -114.8388) (-23.5947, -116.5098) (-28.0082, -116.1359) (-34.3761, -114.2949) (-41.7988, -111.8952) (-49.2951, -109.9846) (-55.9804, -109.5511) (-61.2816, -111.2912) (-64.9891, -115.5355) (-67.1541, -122.3274) (-68.0282, -131.4597) (-67.9856, -142.527) (-67.4559, -154.9716) (-66.846, -168.1309) (-66.4862, -181.285) (-66.6339, -193.707) (-67.4669, -204.7129) (-69.0806, -213.7115) (-71.4836, -220.2539) (-74.5927, -224.0865) (-78.2307, -225.1955) (-82.1162, -223.8722) (-85.8771, -220.7195) (-89.1465, -216.466) (-91.6368, -211.8243) (-93.2381, -207.3088) (-94.0545, -203.1451) (-94.3152, -199.3481) (-94.3152, -195.7677) (-94.337, -192.1417) (-94.5559, -188.9623) (-94.9043, -186.3081) (-95.2266, -184.4038) (-95.4102, -183.4178) knots 0.171909 0.171909 0.171909 0.171909 0.171909 0.171909 0.181818 0.2 0.218182 0.236364 0.254545 0.272727 0.290909 0.309091 0.327273 0.345455 0.363636 0.381818 0.4 0.418182 0.436364 0.454545 0.472727 0.490909 0.509091 0.527273 0.545455 0.563636 0.581818 0.6 0.618182 0.636364 0.654545 0.672727 0.690909 0.709091 0.727273 0.745455 0.763636 0.781818 0.8 0.818182 0.836364 0.854545 0.872727 0.890909 0.909091 0.927273 0.945455 0.963636 0.981818 1 1 1 1 1 1
  line L9 (-67.0516, -49.2025) -> (-70.033, -49.527)
  line L10 (-70.033, -49.527) -> (-70.5018, -45.2191)
  line L11 (-70.5018, -45.2191) -> (-67.5194, -44.8945)
  line L12 (-67.5194, -44.8945) -> (-67.4896, -44.8945)
  spline S4 degree 5 poles (-67.9483, -40.5823) (-67.8539, -41.4324) (-67.7612, -42.2898) (-67.6698, -43.1533) (-67.5794, -44.0219) (-67.4896, -44.8945) knots 0.152948 0.152948 0.152948 0.152948 0.152948 0.152948 0.162519 0.162519 0.162519 0.162519 0.162519 0.162519
  line L13 (-85.6281, -203.631) -> (-82.6737, -204.1519)
  line L14 (-82.6737, -204.1519) -> (-84.4102, -214)
  line L15 (-84.4102, -214) -> (-87.3646, -213.4791)
  line L16 (-87.3646, -213.4791) -> (-85.6281, -203.631)
  line L17 (-47.4308, -202.2827) -> (-47.4308, -211.2827)
  line L18 (-47.4308, -211.2827) -> (-50.4308, -211.2827)
  line L19 (-50.4308, -211.2827) -> (-50.4308, -202.2827)
  line L20 (-50.4308, -202.2827) -> (-47.4308, -202.2827)
  line L21 (-56.2083, -186.8837) -> (-50.2083, -197.276)
  line L22 (-50.2083, -197.276) -> (-52.8064, -198.776)
  line L23 (-52.8064, -198.776) -> (-58.8064, -188.3837)
  line L24 (-58.8064, -188.3837) -> (-56.2083, -186.8837)
  line L25 (-44.8224, -203.3284) -> (-41.84, -203.653)
  line L26 (-41.84, -203.653) -> (-40.4335, -190.7293)
  arc A0 (-40.4335, -190.7293) -> (-46.635, -183.013) centre (-47.3924, -189.972) ccw
  line L27 (-46.635, -183.013) -> (-52.5998, -182.3639)
  arc A1 (-52.5998, -182.3639) -> (-60.3161, -188.5654) centre (-53.3572, -189.3228) ccw
  line L28 (-60.3161, -188.5654) -> (-62.7324, -210.7677)
  arc A2 (-62.7324, -210.7677) -> (-56.5308, -218.4839) centre (-55.7735, -211.525) ccw
  line L29 (-56.5308, -218.4839) -> (-50.566, -219.1331)
  arc A3 (-50.566, -219.1331) -> (-42.8498, -212.9315) centre (-49.8087, -212.1742) ccw
  line L30 (-42.8498, -212.9315) -> (-42.3088, -207.9609)
  line L31 (-42.3088, -207.9609) -> (-45.2912, -207.6363)
  line L32 (-45.2912, -207.6363) -> (-44.8224, -203.3284)
  line L33 (-32.7874, -167.521) -> (-32.7874, -158.521)
  line L34 (-32.7874, -158.521) -> (-29.7874, -158.521)
  line L35 (-29.7874, -158.521) -> (-29.7874, -167.521)
  line L36 (-29.7874, -167.521) -> (-32.7874, -167.521)
  line L37 (-30.01, -153.5144) -> (-24.01, -143.1221)
  line L38 (-24.01, -143.1221) -> (-21.4119, -144.6221)
  line L39 (-21.4119, -144.6221) -> (-27.4119, -155.0144)
  line L40 (-27.4119, -155.0144) -> (-30.01, -153.5144)
  line L41 (-38.3783, -159.8914) -> (-35.3959, -159.5668)
  line L42 (-35.3959, -159.5668) -> (-34.9271, -163.8747)
  line L43 (-34.9271, -163.8747) -> (-37.9095, -164.1993)
  line L44 (-37.9095, -164.1993) -> (-37.3685, -169.1699)
  arc A4 (-37.3685, -169.1699) -> (-29.6522, -175.3715) centre (-30.4096, -168.4126) ccw
  line L45 (-29.6522, -175.3715) -> (-23.6874, -174.7223)
  arc A5 (-23.6874, -174.7223) -> (-17.4859, -167.0061) centre (-24.4448, -167.7634) ccw
  line L46 (-17.4859, -167.0061) -> (-19.9022, -144.8038)
  arc A6 (-19.9022, -144.8038) -> (-27.6185, -138.6023) centre (-26.8611, -145.5612) ccw
  line L47 (-27.6185, -138.6023) -> (-33.5832, -139.2514)
  arc A7 (-33.5832, -139.2514) -> (-39.7848, -146.9677) centre (-32.8259, -146.2103) ccw
  line L48 (-39.7848, -146.9677) -> (-38.3783, -159.8914)
  line L49 (-48.3963, -127.525) -> (-51.3963, -127.525)
  line L50 (-51.3963, -127.525) -> (-51.3963, -131.8584)
  line L51 (-51.3963, -131.8584) -> (-43.3974, -131.8584)
  line L52 (-43.3974, -131.8584) -> (-43.3974, -127.525)
  line L53 (-43.3974, -127.525) -> (-46.4376, -127.525)
  spline S5 degree 5 poles (-46.4376, -127.525) (-46.4394, -126.6696) (-46.4388, -125.8073) (-46.4362, -124.939) (-46.4321, -124.0657) (-46.427, -123.1885) knots 0.152948 0.152948 0.152948 0.152948 0.152948 0.152948 0.162519 0.162519 0.162519 0.162519 0.162519 0.162519
  line L54 (-46.427, -123.1885) -> (-43.3974, -123.1917)
  line L55 (-43.3974, -123.1917) -> (-43.3974, -118.8584)
  line L56 (-43.3974, -118.8584) -> (-51.3963, -118.8584)
  line L57 (-51.3963, -118.8584) -> (-51.3963, -123.1917)
  line L58 (-51.3963, -123.1917) -> (-48.3963, -123.1917)
  line L59 (-48.3963, -123.1917) -> (-48.3963, -127.525)
  line L60 (-39.8042, -85.8319) -> (-36.8042, -85.8319)
  line L61 (-36.8042, -85.8319) -> (-36.8042, -90.1653)
  line L62 (-36.8042, -90.1653) -> (-27.8042, -90.1653)
  line L63 (-27.8042, -90.1653) -> (-27.8042, -85.8319)
  line L64 (-27.8042, -85.8319) -> (-24.8042, -85.8319)
  line L65 (-24.8042, -85.8319) -> (-24.8042, -81.4986)
  line L66 (-24.8042, -81.4986) -> (-27.8042, -81.4986)
  line L67 (-27.8042, -81.4986) -> (-27.8042, -77.1653)
  line L68 (-27.8042, -77.1653) -> (-36.8042, -77.1653)
  line L69 (-36.8042, -77.1653) -> (-36.8042, -81.4986)
  line L70 (-36.8042, -81.4986) -> (-39.8042, -81.4986)
  line L71 (-39.8042, -81.4986) -> (-39.8042, -85.8319)
  line L72 (-23.5469, -21.2767) -> (-26.5469, -21.2767)
  line L73 (-26.5469, -21.2767) -> (-26.5469, -16.9434)
  line L74 (-26.5469, -16.9434) -> (-35.5469, -16.9434)
  line L75 (-35.5469, -16.9434) -> (-35.5469, -21.2767)
  line L76 (-35.5469, -21.2767) -> (-38.5469, -21.2767)
  line L77 (-38.5469, -21.2767) -> (-38.5469, -25.6101)
  line L78 (-38.5469, -25.6101) -> (-35.5469, -25.6101)
  line L79 (-35.5469, -25.6101) -> (-35.5469, -29.9434)
  line L80 (-35.5469, -29.9434) -> (-26.5469, -29.9434)
  line L81 (-26.5469, -29.9434) -> (-26.5469, -25.6101)
  line L82 (-26.5469, -25.6101) -> (-23.5469, -25.6101)
  line L83 (-23.5469, -25.6101) -> (-23.5469, -21.2767)
  line L84 (-57.9052, -26.7992) -> (-60.9052, -26.7992)
  line L85 (-60.9052, -26.7992) -> (-60.9052, -31.1326)
  line L86 (-60.9052, -31.1326) -> (-52.9063, -31.1326)
  line L87 (-52.9063, -31.1326) -> (-52.9063, -26.7992)
  line L88 (-52.9063, -26.7992) -> (-55.9465, -26.7992)
  spline S6 degree 5 poles (-55.9359, -22.4627) (-55.941, -23.3399) (-55.9451, -24.2132) (-55.9477, -25.0815) (-55.9483, -25.9439) (-55.9465, -26.7992) knots -0.162519 -0.162519 -0.162519 -0.162519 -0.162519 -0.162519 -0.152948 -0.152948 -0.152948 -0.152948 -0.152948 -0.152948
  line L89 (-55.9359, -22.4627) -> (-52.9063, -22.4659)
  line L90 (-52.9063, -22.4659) -> (-52.9063, -18.1326)
  line L91 (-52.9063, -18.1326) -> (-60.9052, -18.1326)
  line L92 (-60.9052, -18.1326) -> (-60.9052, -22.4659)
  line L93 (-60.9052, -22.4659) -> (-57.9052, -22.4659)
  line L94 (-57.9052, -22.4659) -> (-57.9052, -26.7992)
  line L95 (-118, -11.8797) -> (-118, -14.8797)
  line L96 (-118, -14.8797) -> (-124, -14.8797)
  line L97 (-124, -14.8797) -> (-124, -11.8797)
  line L98 (-124, -11.8797) -> (-118, -11.8797)
  circle A8 centre (-121, -13.3797) radius 17.5
  line L99 (-134.007, -52.6085) -> (-130.1503, -48.0122)
  line L100 (-130.1503, -48.0122) -> (-142.407, -37.7276)
  line L101 (-142.407, -37.7276) -> (-144.3353, -40.0257)
  line L102 (-144.3353, -40.0257) -> (-148.1656, -36.8118)
  line L103 (-148.1656, -36.8118) -> (-152.0223, -41.4081)
  line L104 (-152.0223, -41.4081) -> (-148.1921, -44.622)
  line L105 (-148.1921, -44.622) -> (-150.1204, -46.9201)
  line L106 (-150.1204, -46.9201) -> (-111.8182, -79.0595)
  line L107 (-111.8182, -79.0595) -> (-109.8899, -76.7614)
  line L108 (-109.8899, -76.7614) -> (-106.0596, -79.9753)
  line L109 (-106.0596, -79.9753) -> (-102.2029, -75.3791)
  line L110 (-102.2029, -75.3791) -> (-106.0331, -72.1651)
  line L111 (-106.0331, -72.1651) -> (-104.1048, -69.867)
  line L112 (-104.1048, -69.867) -> (-116.3615, -59.5824)
  line L113 (-116.3615, -59.5824) -> (-120.2182, -64.1787)
  line L114 (-120.2182, -64.1787) -> (-122.5163, -62.2503)
  line L115 (-122.5163, -62.2503) -> (-118.6596, -57.654)
  line L116 (-118.6596, -57.654) -> (-127.8521, -49.9406)
  line L117 (-127.8521, -49.9406) -> (-131.7089, -54.5368)
  line L118 (-131.7089, -54.5368) -> (-134.007, -52.6085)
  line L119 (-157.101, -20.5868) -> (-160.1234, -20.9153)
  line L120 (-160.1234, -20.9153) -> (-160.5916, -16.6073)
  line L121 (-160.5916, -16.6073) -> (-157.6092, -16.2832)
  spline S7 degree 5 poles (-181.56, -0.0012) (-180.3813, 1.02) (-178.1036, 2.8668) (-174.9263, 5.0504) (-171.1689, 6.7878) (-167.2618, 7.0169) (-164.1162, 5.3522) (-161.6733, 1.8961) (-159.8824, -3.043) (-158.8153, -7.995) (-158.1625, -12.1108) (-157.7796, -14.9403) (-157.6092, -16.2832) knots 0 0 0 0 0 0 0.018182 0.036364 0.054545 0.072727 0.090909 0.109091 0.127273 0.14306 0.14306 0.14306 0.14306 0.14306 0.14306
  spline S8 degree 5 poles (-181.56, -0.0012) (-181.6565, -0.4988) (-181.8645, -1.4865) (-182.2212, -2.946) (-182.7674, -4.8545) (-183.4814, -7.2035) (-183.9988, -9.072) (-184.3147, -10.4749) (-184.4859, -11.4117) (-184.5617, -11.8805) knots 0 0 0 0 0 0 0.2 0.4 0.6 0.8 1 1 1 1 1 1
  line L122 (-184.5617, -11.8805) -> (-178.5617, -11.8813)
  line L123 (-178.5617, -11.8813) -> (-178.5621, -14.8813)
  line L124 (-178.5621, -14.8813) -> (-184.5621, -14.8805)
  spline S9 degree 5 poles (-184.5621, -14.8805) (-185.7139, -22.3102) (-187.6822, -36.704) (-189.6298, -56.899) (-190.4936, -81.4163) (-189.6467, -109.3683) (-188.0181, -130.3755) (-186.433, -145.5955) (-185.2244, -155.5154) (-184.5821, -160.4186) knots 0 0 0 0 0 0 0.2 0.4 0.6 0.8 1 1 1 1 1 1
  line L125 (-184.5821, -160.4186) -> (-178.5821, -160.4194)
  line L126 (-178.5821, -160.4194) -> (-178.5826, -163.4194)
  line L127 (-178.5826, -163.4194) -> (-184.5826, -163.4186)
  spline S10 degree 5 poles (-156.2055, -29.2072) (-156.1131, -30.12) (-155.8503, -32.7099) (-155.4078, -36.9682) (-154.7411, -42.7674) (-153.7249, -49.6128) (-152.3127, -55.9588) (-150.5146, -60.8114) (-148.2312, -64.0978) (-145.3471, -66.0564) (-141.7155, -67.3506) (-137.2316, -68.8476) (-131.931, -71.3259) (-126.0635, -75.2392) (-120.2164, -80.3793) (-115.207, -86.0005) (-111.8825, -91.1333) (-110.9397, -94.8497) (-112.7578, -96.5204) (-117.1713, -96.146) (-123.5389, -94.3041) (-130.9613, -91.9034) (-138.4573, -89.9917) (-145.1426, -89.5573) (-150.444, -91.2967) (-154.1521, -95.5404) (-156.318, -102.332) (-157.1934, -111.4642) (-157.1523, -122.5315) (-156.6243, -134.9762) (-156.0163, -148.1356) (-155.6583, -161.2897) (-155.8076, -173.7117) (-156.6422, -184.7175) (-158.2571, -193.7158) (-160.661, -200.258) (-163.7707, -204.0901) (-167.4088, -205.1986) (-171.2941, -203.8748) (-175.0546, -200.7216) (-178.3234, -196.4676) (-180.8131, -191.8255) (-182.4137, -187.3098) (-183.2295, -183.146) (-183.4898, -179.349) (-183.4893, -175.7686) (-183.5106, -172.1426) (-183.729, -168.9631) (-184.0771, -166.3089) (-184.3991, -164.4045) (-184.5826, -163.4186) knots 0.171909 0.171909 0.171909 0.171909 0.171909 0.171909 0.181818 0.2 0.218182 0.236364 0.254545 0.272727 0.290909 0.309091 0.327273 0.345455 0.363636 0.381818 0.4 0.418182 0.436364 0.454545 0.472727 0.490909 0.509091 0.527273 0.545455 0.563636 0.581818 0.6 0.618182 0.636364 0.654545 0.672727 0.690909 0.709091 0.727273 0.745455 0.763636 0.781818 0.8 0.818182 0.836364 0.854545 0.872727 0.890909 0.909091 0.927273 0.945455 0.963636 0.981818 1 1 1 1 1 1
  line L128 (-156.2055, -29.2072) -> (-159.1869, -29.5312)
  line L129 (-159.1869, -29.5312) -> (-159.6551, -25.2233)
  line L130 (-159.6551, -25.2233) -> (-156.6727, -24.8991)
  line L131 (-156.6727, -24.8991) -> (-156.6428, -24.8991)
  spline S11 degree 5 poles (-157.101, -20.5868) (-157.0067, -21.437) (-156.9142, -22.2944) (-156.8229, -23.1579) (-156.7325, -24.0265) (-156.6428, -24.8991) knots 0.152948 0.152948 0.152948 0.152948 0.152948 0.152948 0.162519 0.162519 0.162519 0.162519 0.162519 0.162519
  line L132 (-174.8033, -183.6331) -> (-171.8489, -184.1544)
  line L133 (-171.8489, -184.1544) -> (-173.5868, -194.0023)
  line L134 (-173.5868, -194.0023) -> (-176.5411, -193.4809)
  line L135 (-176.5411, -193.4809) -> (-174.8033, -183.6331)
  line L136 (-213, -16.8797) -> (-213, -19.8797)
  line L137 (-213, -19.8797) -> (-219, -19.8797)
  line L138 (-219, -19.8797) -> (-219, -16.8797)
  line L139 (-219, -16.8797) -> (-213, -16.8797)
  circle A9 centre (-216, -18.3797) radius 17.5
  line L140 (-199.9121, -50.3584) -> (-241.9121, -50.3584)
  line L141 (-241.9121, -50.3584) -> (-241.9121, -59.3584)
  line L142 (-241.9121, -59.3584) -> (-199.9121, -59.3584)
  line L143 (-199.9121, -59.3584) -> (-199.9121, -50.3584)
  line L144 (-200.5488, -94.516) -> (-200.5488, -82.516)
  line L145 (-200.5488, -82.516) -> (-242.5488, -82.516)
  line L146 (-242.5488, -82.516) -> (-242.5488, -94.516)
  line L147 (-242.5488, -94.516) -> (-200.5488, -94.516)
  line L148 (-202, -109.1519) -> (-240, -109.1519)
  line L149 (-240, -109.1519) -> (-240, -119.1519)
  line L150 (-240, -119.1519) -> (-202, -119.1519)
  line L151 (-202, -119.1519) -> (-202, -109.1519)
  line L152 (-126, -160.4178) -> (-126, -163.4178)
  line L153 (-126, -163.4178) -> (-132, -163.4178)
  line L154 (-132, -163.4178) -> (-132, -160.4178)
  line L155 (-132, -160.4178) -> (-126, -160.4178)
  circle A10 centre (-129, -161.9178) radius 17.5
  line L156 (-227, -163.4178) -> (-227, -160.4178)
  line L157 (-227, -160.4178) -> (-221, -160.4178)
  line L158 (-221, -160.4178) -> (-221, -163.4178)
  line L159 (-221, -163.4178) -> (-227, -163.4178)
  circle A11 centre (-224, -161.9178) radius 17.5
  line L160 (-148.3509, -108.1309) -> (-144.5207, -111.3448)
  line L161 (-144.5207, -111.3448) -> (-146.449, -113.643)
  line L162 (-146.449, -113.643) -> (-115.8073, -139.3545)
  line L163 (-115.8073, -139.3545) -> (-113.8789, -137.0563)
  line L164 (-113.8789, -137.0563) -> (-110.0487, -140.2703)
  line L165 (-110.0487, -140.2703) -> (-106.192, -135.674)
  line L166 (-106.192, -135.674) -> (-110.0222, -132.4601)
  line L167 (-110.0222, -132.4601) -> (-108.0938, -130.1619)
  line L168 (-108.0938, -130.1619) -> (-116.5203, -123.0913)
  line L169 (-116.5203, -123.0913) -> (-120.377, -127.6875)
  line L170 (-120.377, -127.6875) -> (-122.6752, -125.7592)
  line L171 (-122.6752, -125.7592) -> (-118.8184, -121.1629)
  line L172 (-118.8184, -121.1629) -> (-128.011, -113.4495)
  line L173 (-128.011, -113.4495) -> (-131.8677, -118.0457)
  line L174 (-131.8677, -118.0457) -> (-134.1658, -116.1174)
  line L175 (-134.1658, -116.1174) -> (-130.3091, -111.5211)
  line L176 (-130.3091, -111.5211) -> (-138.7356, -104.4504)
  line L177 (-138.7356, -104.4504) -> (-140.664, -106.7486)
  line L178 (-140.664, -106.7486) -> (-144.4942, -103.5346)
  line L179 (-144.4942, -103.5346) -> (-148.3509, -108.1309)